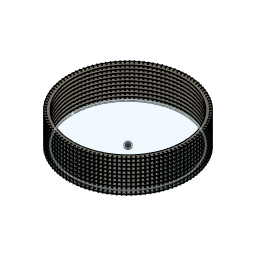
Display v3 (Autodesk Fusion 360 design; units mm, degrees)
Autodesk Fusion 360 part; units mm, degrees
sketch "Sketch1" plane through (0, 0, 0) normal (0, 1, 0) x (1, 0, 0)
  circle A0 centre (0, 0) radius 292
  dimension "d1" = 584
  constraint coincident A0.centre origin
  measures "d1" diameter of A0
extrude "Extrude1" add sketch "Sketch1" along normal blind 3 makes body 1
sketch "Sketch2" plane through (0, 3, 0) normal (0, 1, 0) x (-1, 0, 0)
  circle A0 centre (0, 0) radius 292
  circle A1 centre (0, 0) radius 269.5
  dimension "d4" = 539
  constraint coincident A0.centre A1.centre
  measures "d4" diameter of A1
extrude "Extrude2" cut sketch "Sketch2" against normal up to surface (3 mm away) contours A1 bodies 1
pattern_linear "R-Pattern1" count 10 spacing 16.667 along (0, 1, 0) of bodies 1 makes body 2 at (282.4095, 16.667, 27.8957) makes body 3 at (282.4095, 33.334, 27.8957) makes body 4 at (282.4095, 50.001, 27.8957) makes body 5 at (282.4095, 66.668, 27.8957) makes body 6 at (282.4095, 83.335, 27.8957) makes body 7 at (282.4095, 100.002, 27.8957) makes body 8 at (282.4095, 116.669, 27.8957) makes body 9 at (282.4095, 133.336, 27.8957) makes body 10 at (282.4095, 150.003, 27.8957)
sketch "Sketch3" plane through (0, 0, 0) normal (0, 0, 1) x (1, 0, 0)
  line L0 (292, 156.003) -> (282, 156.003)
  line L1 (282, 156.003) -> (282, -3)
  line L2 (282, -3) -> (292, -3)
  line L3 (292, -3) -> (292, 156.003)
  line L4 (292, 153.003) -> (-292, 153.003)
  line L5 (292, 0) -> (-292, 0)
  point P0 (0, 3)
  dimension "d16" = 10
  dimension "d18" = 3
  dimension "d19" = 3
  dimension "d22" = 292
  constraint horizontal L0
  constraint vertical L1
  constraint horizontal L2
  constraint vertical L3
  constraint coincident L0.end L1.start
  constraint coincident L1.end L2.start
  measures "d16" distance of L1 L3
  measures "d18" distance of L2 L5
  measures "d19" distance of L0 L4
  measures "d22" distance of L3 P0
extrude "Extrude3" add sketch "Sketch3" along normal blind 3 separate body makes body 11
pattern_circular "C-Pattern1" count 110 over 360 about axis through (0, 1.75, 0) along (0, 1, 0) of bodies 11 makes body 12 at (284.868, 102.002, -16.2893) makes body 13 at (283.4735, 102.002, -32.5255) makes body 14 at (281.1543, 102.002, -48.6557) makes body 15 at (277.9181, 102.002, -64.6271) makes body 16 at (273.7753, 102.002, -80.3877) makes body 17 at (268.7396, 102.002, -95.8861) makes body 18 at (262.8273, 102.002, -111.0717) makes body 19 at (256.0577, 102.002, -125.8951) makes body 20 at (248.4529, 102.002, -140.3078) makes body 21 at (240.0377, 102.002, -154.2628) makes body 22 at (230.8395, 102.002, -167.7147) makes body 23 at (220.8884, 102.002, -180.6196) makes body 24 at (210.2168, 102.002, -192.9352) makes body 25 at (198.8595, 102.002, -204.6216) makes body 26 at (186.8536, 102.002, -215.6405) makes body 27 at (174.2382, 102.002, -225.9561) makes body 28 at (161.0545, 102.002, -235.5346) makes body 29 at (147.3454, 102.002, -244.3449) makes body 30 at (133.1557, 102.002, -252.3582) makes body 31 at (118.5318, 102.002, -259.5483) makes body 32 at (103.5211, 102.002, -265.8919) makes body 33 at (88.1728, 102.002, -271.3681) makes body 34 at (72.537, 102.002, -275.9592) makes body 35 at (56.6645, 102.002, -279.6502) makes body 36 at (40.6072, 102.002, -282.4291) makes body 37 at (24.4174, 102.002, -284.2867) makes body 38 at (8.148, 102.002, -285.217) makes body 39 at (-8.148, 102.002, -285.217) makes body 40 at (-24.4174, 102.002, -284.2867) makes body 41 at (-40.6072, 102.002, -282.4291) makes body 42 at (-56.6645, 102.002, -279.6502) makes body 43 at (-72.537, 102.002, -275.9592) makes body 44 at (-88.1728, 102.002, -271.3681) makes body 45 at (-103.5211, 102.002, -265.8919) makes body 46 at (-118.5318, 102.002, -259.5483) makes body 47 at (-133.1557, 102.002, -252.3582) makes body 48 at (-147.3454, 102.002, -244.3449) makes body 49 at (-161.0545, 102.002, -235.5346) makes body 50 at (-174.2382, 102.002, -225.9561) makes body 51 at (-186.8536, 102.002, -215.6405) makes body 52 at (-198.8595, 102.002, -204.6216) makes body 53 at (-210.2168, 102.002, -192.9352) makes body 54 at (-220.8884, 102.002, -180.6196) makes body 55 at (-230.8395, 102.002, -167.7147) makes body 56 at (-240.0377, 102.002, -154.2628) makes body 57 at (-248.4529, 102.002, -140.3078) makes body 58 at (-256.0577, 102.002, -125.8951) makes body 59 at (-262.8273, 102.002, -111.0717) makes body 60 at (-268.7396, 102.002, -95.8861) makes body 61 at (-273.7753, 102.002, -80.3877) makes body 62 at (-277.9181, 102.002, -64.6271) makes body 63 at (-281.1543, 102.002, -48.6557) makes body 64 at (-283.4735, 102.002, -32.5255) makes body 65 at (-284.868, 102.002, -16.2893) makes body 66 at (-285.3333, 102.002, 0) makes body 67 at (-284.868, 102.002, 16.2893) makes body 68 at (-283.4735, 102.002, 32.5255) makes body 69 at (-281.1543, 102.002, 48.6557) makes body 70 at (-277.9181, 102.002, 64.6271) makes body 71 at (-273.7753, 102.002, 80.3877) makes body 72 at (-268.7396, 102.002, 95.8861) makes body 73 at (-262.8273, 102.002, 111.0717) makes body 74 at (-256.0577, 102.002, 125.8951) makes body 75 at (-248.4529, 102.002, 140.3078) makes body 76 at (-240.0377, 102.002, 154.2628) makes body 77 at (-230.8395, 102.002, 167.7147) makes body 78 at (-220.8884, 102.002, 180.6196) makes body 79 at (-210.2168, 102.002, 192.9352) makes body 80 at (-198.8595, 102.002, 204.6216) makes body 81 at (-186.8536, 102.002, 215.6405) makes body 82 at (-174.2382, 102.002, 225.9561) makes body 83 at (-161.0545, 102.002, 235.5346) makes body 84 at (-147.3454, 102.002, 244.3449) makes body 85 at (-133.1557, 102.002, 252.3582) makes body 86 at (-118.5318, 102.002, 259.5483) makes body 87 at (-103.5211, 102.002, 265.8919) makes body 88 at (-88.1728, 102.002, 271.3681) makes body 89 at (-72.537, 102.002, 275.9592) makes body 90 at (-56.6645, 102.002, 279.6502) makes body 91 at (-40.6072, 102.002, 282.4291) makes body 92 at (-24.4174, 102.002, 284.2867) makes body 93 at (-8.148, 102.002, 285.217) makes body 94 at (8.148, 102.002, 285.217) makes body 95 at (24.4174, 102.002, 284.2867) makes body 96 at (40.6072, 102.002, 282.4291) makes body 97 at (56.6645, 102.002, 279.6502) makes body 98 at (72.537, 102.002, 275.9592) makes body 99 at (88.1728, 102.002, 271.3681) makes body 100 at (103.5211, 102.002, 265.8919) makes body 101 at (118.5318, 102.002, 259.5483) makes body 102 at (133.1557, 102.002, 252.3582) makes body 103 at (147.3454, 102.002, 244.3449) makes body 104 at (161.0545, 102.002, 235.5346) makes body 105 at (174.2382, 102.002, 225.9561) makes body 106 at (186.8536, 102.002, 215.6405) makes body 107 at (198.8595, 102.002, 204.6216) makes body 108 at (210.2168, 102.002, 192.9352) makes body 109 at (220.8884, 102.002, 180.6196) makes body 110 at (230.8395, 102.002, 167.7147) makes body 111 at (240.0377, 102.002, 154.2628) makes body 112 at (248.4529, 102.002, 140.3078) makes body 113 at (256.0577, 102.002, 125.8951) makes body 114 at (262.8273, 102.002, 111.0717) makes body 115 at (268.7396, 102.002, 95.8861) makes body 116 at (273.7753, 102.002, 80.3877) makes body 117 at (277.9181, 102.002, 64.6271) makes body 118 at (281.1543, 102.002, 48.6557) makes body 119 at (283.4735, 102.002, 32.5255) makes body 120 at (284.868, 102.002, 16.2893)
copy_body "CutPasteBodies1" bodies 1 9 8 10 6 2 7 5 3 4 removing the originals makes body 121 makes body 122 makes body 123 makes body 124 makes body 125 makes body 126 makes body 127 makes body 128 makes body 129 makes body 130 in component "Circles"
copy_body "CutPasteBodies1'" bodies 120 54 45 56 41 39 52 57 38 36 42 46 47 50 44 51 55 37 40 43 48 49 53 66 74 75 76 79 71 58 64 69 72 77 78 62 61 59 63 60 65 67 68 70 73 86 93 84 94 95 97 98 85 92 91 81 99 87 100 101 88 80 96 83 82 89 90 111 114 116 103 104 105 108 109 102 117 118 113 107 110 119 106 112 115 35 34 29 31 28 33 30 32 26 27 19 25 16 15 17 18 20 14 21 22 23 24 12 13 11 removing the originals makes body 131 makes body 132 makes body 133 makes body 134 makes body 135 makes body 136 makes body 137 makes body 138 makes body 139 makes body 140 makes body 141 makes body 142 makes body 143 makes body 144 makes body 145 makes body 146 makes body 147 makes body 148 makes body 149 makes body 150 makes body 151 makes body 152 makes body 153 makes body 154 makes body 155 makes body 156 makes body 157 makes body 158 makes body 159 makes body 160 makes body 161 makes body 162 makes body 163 makes body 164 makes body 165 makes body 166 makes body 167 makes body 168 makes body 169 makes body 170 makes body 171 makes body 172 makes body 173 makes body 174 makes body 175 makes body 176 makes body 177 makes body 178 makes body 179 makes body 180 makes body 181 makes body 182 makes body 183 makes body 184 makes body 185 makes body 186 makes body 187 makes body 188 makes body 189 makes body 190 makes body 191 makes body 192 makes body 193 makes body 194 makes body 195 makes body 196 makes body 197 makes body 198 makes body 199 makes body 200 makes body 201 makes body 202 makes body 203 makes body 204 makes body 205 makes body 206 makes body 207 makes body 208 makes body 209 makes body 210 makes body 211 makes body 212 makes body 213 makes body 214 makes body 215 makes body 216 makes body 217 makes body 218 makes body 219 makes body 220 makes body 221 makes body 222 makes body 223 makes body 224 makes body 225 makes body 226 makes body 227 makes body 228 makes body 229 makes body 230 makes body 231 makes body 232 makes body 233 makes body 234 makes body 235 makes body 236 makes body 237 makes body 238 makes body 239 makes body 240 in component "Slots"
component "Circles" placed x (1, 0, 0) y (0, 1, 0) z (0, 0, 1) at (0, 0, 0)
component "Slots" placed x (1, 0, 0) y (0, 1, 0) z (0, 0, 1) at (0, 0, 0)
named bodies: "Circle1", "Circle2", "Slot1", "Slot1 (1)", "Slot1 (2)", "Slot1 (3)", "Slot1 (4)", "Slot1 (5)", "Slot1 (6)", "Slot1 (7)", "Slot1 (8)", "Slot1 (9)", "Slot1 (10)", "Slot1 (11)", "Slot1 (12)", "Slot1 (13)", "Slot1 (14)", "Slot1 (15)", "Slot1 (16)", "Slot1 (17)", "Slot1 (18)", "Slot1 (19)", "Slot1 (20)", "Slot1 (21)", "Slot1 (22)", "Slot1 (23)", "Slot1 (24)", "Slot1 (25)", "Slot1 (26)", "Slot1 (27)", "Slot1 (28)", "Slot1 (29)", "Slot1 (30)", "Slot1 (31)", "Slot1 (32)", "Slot1 (33)", "Slot1 (34)", "Slot1 (35)", "Slot1 (36)", "Slot1 (37)", "Slot1 (38)", "Slot1 (39)", "Slot1 (40)", "Slot1 (41)", "Slot1 (42)", "Slot1 (43)", "Slot1 (44)", "Slot1 (45)", "Slot1 (46)", "Slot1 (47)", "Slot1 (48)", "Slot1 (49)", "Slot1 (50)", "Slot1 (51)", "Slot1 (52)", "Slot1 (53)", "Slot1 (54)", "Slot1 (55)", "Slot1 (56)", "Slot1 (57)", "Slot1 (58)", "Slot1 (59)", "Slot1 (60)", "Slot1 (61)", "Slot1 (62)", "Slot1 (63)", "Slot1 (64)", "Slot1 (65)", "Slot1 (66)", "Slot1 (67)", "Slot1 (68)", "Slot1 (69)", "Slot1 (70)", "Slot1 (71)", "Slot1 (72)", "Slot1 (73)", "Slot1 (74)", "Slot1 (75)", "Slot1 (76)", "Slot1 (77)", "Slot1 (78)", "Slot1 (79)", "Slot1 (80)", "Slot1 (81)", "Slot1 (82)", "Slot1 (83)", "Slot1 (84)", "Slot1 (85)", "Slot1 (86)", "Slot1 (87)", "Slot1 (88)", "Slot1 (89)", "Slot1 (90)", "Slot1 (91)", "Slot1 (92)", "Slot1 (93)", "Slot1 (94)", "Slot1 (95)", "Slot1 (96)", "Slot1 (97)", "Slot1 (98)", "Slot1 (99)", "Slot1 (100)", "Slot1 (101)", "Slot1 (102)", "Slot1 (103)", "Slot1 (104)", "Slot1 (105)", "Slot1 (106)", "Slot1 (107)", "Slot1 (108)", "Slot1 (109)"
